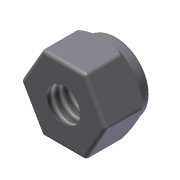
# Autodesk Inventor part: 14-20 regular lock nut
Saved by Autodesk Inventor 2013 (Build 170138000, 138)
## iProperties
Created: 2011-07-10
Part Number: 14-20 regular lock nut
Document SubType Name: Modeling
Designer: Dan Niemitalo
Density: 5.81972 g/cm^3
Material: Steel
Mass: 3.719 g
Surface Area: 5.94086 cm^2
Volume: 0.639034 cm^3
Author: Dan Niemitalo
Autodesk Inventor part; units mm, degrees
ref_plane "YZ Plane" through (0, 0, 0) normal (1, 0, 0) x (0, 1, 0)
ref_plane "XZ Plane" through (0, 0, 0) normal (0, 1, 0) x (-1, 0, 0)
ref_plane "XY Plane" through (0, 0, 0) normal (0, 0, 1) x (1, 0, 0)
sketch "Sketch1" plane through (0, 0, 0) normal (0, 0, 1) x (1, 0, 0)
  line L0 (-3.2079, 5.5563) -> (3.2079, 5.5563)
  line L1 (3.2079, 5.5563) -> (6.4158, 0)
  line L2 (6.4158, 0) -> (3.2079, -5.5563)
  line L3 (3.2079, -5.5563) -> (-3.2079, -5.5562)
  line L4 (-3.2079, -5.5562) -> (-6.4158, 0)
  line L5 (-6.4158, 0) -> (-3.2079, 5.5563)
  point P0 (0, 0)
  point P1 (0, 0)
  dimension "d0" = 11.1125
  constraints: 12 end point, 1 coincident, 1 horizontal, 13 other
  measures "d0" distance between parallel lines of L3 L0
extrude "Extrusion1" add sketch "Sketch1" along normal blind 6.35
sketch "Sketch3" plane through (0, 0, 6.35) normal (0, 0, 1) x (1, 0, 0)
  circle A0 centre (0, 0) radius 5.08
  dimension "d28" = 10.16
  constraints: 1 centre point, 1 coincident
  measures "d28" diameter of A0
extrude "Extrusion2" add sketch "Sketch3" along normal blind 1.5875
sketch "Sketch8" plane through (0, 0, 7.9375) normal (0, 0, 1) x (1, 0, 0)
  circle A0 centre (0, 0) radius 5.08 projected
  circle A1 centre (0, 0) radius 3.175
  dimension "d29" = 6.35
  constraints: 1 centre point, 1 coincident
  measures "d29" diameter of A1
sketch "Sketch9" plane through (0, 0, 0) normal (0, 0, -1) x (-1, 0, 0)
  point P0 (0, 0)
hole "Hole2" at (0, 0, 0) direction (0, 0, 1) diameter 4.9784 end through all thread size "1/4-20 UNC" class "2B" standard "ANSI Unified Screw Threads"
sketch "Sketch10" plane through (0, 0, 0) normal (0, 1, 0) x (-1, 0, 0)
  line L0 (-6.4158, 6.35) -> (-3.2079, 6.35) projected
  line L1 (-3.2079, 0) -> (-3.2079, 6.35) projected
  line L2 (-6.4158, 0) -> (-3.2079, 0) projected
  line L3 (-6.4158, 0) -> (-6.4158, 6.35) projected
  line L4 (0, 0) -> (0, 6.9243)
  arc A0 (-4.572, 6.35) -> (-6.4158, 5.1517) centre (-4.572, 4.3324) ccw
  line L5 (-6.4158, 5.1517) -> (-6.4158, 6.35)
  line L6 (-4.572, 6.35) -> (-6.4158, 6.35)
  dimension "d24" = 4.572
  constraints: 6 end point, 2 parallel, 2 point on circle, 2 point on line, 2 tangent, 1 centre point, 1 collinear
  measures "d24" distance from line of L4 L6.start
revolve "Revolution2" cut sketch "Sketch10" angle 360 about axis through (0, 0, 0) along (0, 0, 1) contours L0 A0 L3
fillet "Fillet1" radius 0.508 12 edges at (-3.2079, -5.5562, 2.5758) (3.2079, -5.5563, 2.5758) (6.4158, 0, 2.5758) (3.2079, 5.5563, 2.5758) (-6.4158, 0, 2.5758) (-3.2079, 5.5563, 2.5758) (0, 5.5563, 0) (4.8119, 2.7781, 0) (4.8119, -2.7781, 0) (0, -5.5563, 0) (-4.8119, -2.7781, 0) (-4.8119, 2.7781, 0)
fillet "Fillet2" radius 0.508 1 edges at (-5.08, 0, 7.9375)
extrude "Extrusion4" cut sketch "Sketch8" against normal blind 0.254 contours A1
body "Solid1"
